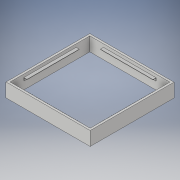
# Autodesk Inventor part: Bumper
Saved by Autodesk Inventor 2018 (Build 220112000, 112)
## iProperties
Created: 2019-02-23
Part Number: Bumper
Material: Generic
Document SubType Name: Modeling
Designer: s-2513226
Density: 1 g/cm^3
Appearance: Default
Author: s-2513226
Autodesk Inventor part; units mm, degrees
ref_plane "YZ Plane" through (0, 0, 0) normal (1, 0, 0) x (0, 1, 0)
ref_plane "XZ Plane" through (0, 0, 0) normal (0, 1, 0) x (-1, 0, 0)
ref_plane "XY Plane" through (0, 0, 0) normal (0, 0, 1) x (1, 0, 0)
sketch "Sketch15" plane through (0, 0, 0) normal (0, 1, 0) x (-1, 0, 0)
  line L0 (-369.8875, -368.1356) -> (369.8875, -368.1356)
  line L1 (369.8875, -368.1356) -> (369.8875, 368.4644)
  line L2 (369.8875, 368.4644) -> (-369.8875, 368.4644)
  line L3 (-369.8875, 368.4644) -> (-369.8875, -368.1356)
  line L4 (-389.0391, -387.2872) -> (389.0391, -387.2872)
  line L5 (389.0391, -387.2872) -> (389.0391, 387.616)
  line L6 (389.0391, 387.616) -> (-389.0391, 387.616)
  line L7 (-389.0391, 387.616) -> (-389.0391, -387.2872)
  dimension "d84" = 736.6
  dimension "d85" = 739.775
  dimension "d86" = 19.1516
  dimension "d87" = 19.1516
  dimension "d88" = 19.1516
  dimension "d89" = 19.1516
  constraints: 16 end point, 4 parallel, 2 horizontal, 2 perpendicular
  measures "d84" distance of L0.end L1.end
  measures "d85" distance of L1.end L2.end
  measures "d86" distance between parallel lines of L1 L5
  measures "d87" distance between parallel lines of L2 L6
  measures "d88" distance between parallel lines of L4 L0
  measures "d89" distance between parallel lines of L7 L3
extrude "Extrusion12" add sketch "Sketch15" along normal blind 127
sketch "Sketch16" plane through (-369.8875, 0, -368.1356) normal (1, 0, 0) x (0, 0, -1)
  line L0 (-609.6, 73.66) -> (-127, 73.66)
  line L1 (-127, 73.66) -> (-127, 99.06)
  line L2 (-127, 99.06) -> (-609.6, 99.06)
  line L3 (-609.6, 99.06) -> (-609.6, 73.66)
  line L4 (-736.6, 0) -> (-736.6, 127) projected
  line L5 (0, 0) -> (0, 127) projected
  line L6 (0, 0) -> (-736.6, 0) projected
  point P0 (-368.1356, 0)
  dimension "d92" = 127
  dimension "d93" = 127
  dimension "d94" = 73.66
  dimension "d95" = 25.4
  constraints: 8 end point, 2 parallel, 1 horizontal, 1 perpendicular
  measures "d92" distance between parallel lines of L4 L3
  measures "d93" distance between parallel lines of L5 L1
  measures "d94" distance between parallel lines of L6 L0
  measures "d95" distance of L2.end L0.start
sketch "Sketch17" plane through (-369.8875, 0, -368.1356) normal (0, 0, 1) x (1, 0, 0)
  line L0 (127, 73.66) -> (612.775, 73.66)
  line L1 (612.775, 73.66) -> (612.775, 99.06)
  line L2 (612.775, 99.06) -> (127, 99.06)
  line L3 (127, 99.06) -> (127, 73.66)
  line L4 (0, 0) -> (0, 127) projected
  line L5 (739.775, 0) -> (739.775, 127) projected
  line L6 (739.775, 0) -> (0, 0) projected
  point P0 (369.8875, 0)
  dimension "d96" = 127
  dimension "d97" = 127
  dimension "d98" = 25.4
  dimension "d99" = 73.66
  constraints: 8 end point, 2 parallel, 1 horizontal, 1 perpendicular
  measures "d96" distance between parallel lines of L4 L3
  measures "d97" distance between parallel lines of L5 L1
  measures "d98" distance of L0.end L1.end
  measures "d99" distance between parallel lines of L6 L0
sketch "Sketch18" plane through (369.8875, 0, 368.4644) normal (-1, 0, 0) x (0, 0, 1)
  line L0 (-609.6, 73.66) -> (-127, 73.66)
  line L1 (-127, 73.66) -> (-127, 99.06)
  line L2 (-127, 99.06) -> (-609.6, 99.06)
  line L3 (-609.6, 99.06) -> (-609.6, 73.66)
  line L4 (-736.6, 0) -> (-736.6, 127) projected
  line L5 (0, 0) -> (0, 127) projected
  line L6 (0, 0) -> (-736.6, 0) projected
  point P0 (-368.4644, 0)
  dimension "d100" = 127
  dimension "d101" = 127
  dimension "d102" = 25.4
  dimension "d103" = 73.66
  constraints: 8 end point, 2 parallel, 1 horizontal, 1 perpendicular
  measures "d100" distance between parallel lines of L4 L3
  measures "d101" distance between parallel lines of L5 L1
  measures "d102" distance of L0.end L1.end
  measures "d103" distance between parallel lines of L6 L0
sketch "Sketch19" plane through (369.8875, 0, 368.4644) normal (0, 0, -1) x (-1, 0, 0)
  line L0 (127, 73.66) -> (612.775, 73.66)
  line L1 (612.775, 73.66) -> (612.775, 99.06)
  line L2 (612.775, 99.06) -> (127, 99.06)
  line L3 (127, 99.06) -> (127, 73.66)
  line L4 (739.775, 0) -> (739.775, 127) projected
  line L5 (739.775, 0) -> (0, 0) projected
  point P0 (369.8875, 0)
  point P1 (0, 127)
  dimension "d104" = 127
  dimension "d105" = 127
  dimension "d106" = 25.4
  dimension "d107" = 73.66
  constraints: 8 end point, 2 parallel, 1 horizontal, 1 perpendicular
  measures "d104" distance from line of point (0, 127) L3
  measures "d105" distance between parallel lines of L4 L1
  measures "d106" distance of L0.end L1.end
  measures "d107" distance between parallel lines of L5 L0
extrude "Extrusion13" add sketch "Sketch19" along normal blind 3.175
extrude "Extrusion14" add sketch "Sketch16" along normal blind 3.175
extrude "Extrusion15" add sketch "Sketch18" along normal blind 3.175
extrude "Extrusion16" add sketch "Sketch17" along normal blind 3.175
sketch "Sketch20" plane through (-369.8875, 0, -364.9606) normal (0, 0, 1) x (1, 0, 0)
  line L0 (612.775, 99.06) -> (127, 99.06) projected
  line L1 (127, 99.06) -> (127, 73.66) projected
  line L2 (612.775, 99.06) -> (127, 99.06)
  line L3 (127, 99.06) -> (127, 95.885)
  line L4 (127, 95.885) -> (612.775, 95.885)
  line L5 (612.775, 95.885) -> (612.775, 99.06)
  point P0 (369.8875, 0)
  dimension "d116" = 3.175
  constraints: 8 end point, 2 parallel, 1 horizontal, 1 perpendicular, 1 point on line
  measures "d116" distance of L4.end L0.start
extrude "Extrusion17" add sketch "Sketch20" along normal blind 25.4
sketch "Sketch21" plane through (366.7125, 0, 368.4644) normal (-1, 0, 0) x (0, 0, 1)
  line L0 (-609.6, 99.06) -> (-127, 99.06) projected
  line L1 (-609.6, 99.06) -> (-609.6, 73.66) projected
  line L2 (-127, 99.06) -> (-609.6, 99.06)
  line L3 (-609.6, 99.06) -> (-609.6, 95.885)
  line L4 (-609.6, 95.885) -> (-127, 95.885)
  line L5 (-127, 95.885) -> (-127, 99.06)
  point P0 (-368.4644, 0)
  dimension "d119" = 3.175
  constraints: 8 end point, 2 parallel, 1 horizontal, 1 perpendicular, 1 point on line
  measures "d119" distance of L4.end L0.end
sketch "Sketch22" plane through (369.8875, 0, 365.2894) normal (0, 0, -1) x (-1, 0, 0)
  line L0 (612.775, 73.66) -> (612.775, 99.06) projected
  line L1 (127, 99.06) -> (612.775, 99.06)
  line L2 (612.775, 99.06) -> (612.775, 95.885)
  line L3 (612.775, 95.885) -> (127, 95.885)
  line L4 (127, 95.885) -> (127, 99.06)
  point P0 (369.8875, 0)
  dimension "d120" = 3.175
  constraints: 8 end point, 2 parallel, 1 horizontal, 1 perpendicular, 1 point on line
  measures "d120" distance of L3.end L1.start
extrude "Extrusion18" add sketch "Sketch22" along normal blind 25.4
extrude "Extrusion19" add sketch "Sketch21" along normal blind 25.4
sketch "Sketch23" plane through (-366.7125, 0, -368.1356) normal (1, 0, 0) x (0, 0, -1)
  line L0 (-609.6, 99.06) -> (-127, 99.06) projected
  line L1 (-127, 99.06) -> (-127, 73.66) projected
  line L2 (-609.6, 99.06) -> (-127, 99.06)
  line L3 (-127, 99.06) -> (-127, 95.885)
  line L4 (-127, 95.885) -> (-609.6, 95.885)
  line L5 (-609.6, 95.885) -> (-609.6, 99.06)
  point P0 (-368.1356, 0)
  dimension "d125" = 3.175
  constraints: 8 end point, 2 parallel, 1 horizontal, 1 perpendicular, 1 point on line
  measures "d125" distance of L4.end L0.start
extrude "Extrusion20" add sketch "Sketch23" along normal blind 25.4
equation "\"d87\" = d86"
equation "\"d88\" = d86"
equation "\"d89\" = d86"
equation "\"d93\" = d92"
equation "\"d96\" = d92"
equation "\"d97\" = d92"
equation "\"d100\" = d92"
equation "\"d101\" = d92"
equation "\"d104\" = d92"
equation "\"d105\" = d92"
equation "\"d119\" = d116"
equation "\"d120\" = d116"
equation "\"d125\" = d116"
body "Solid2"
